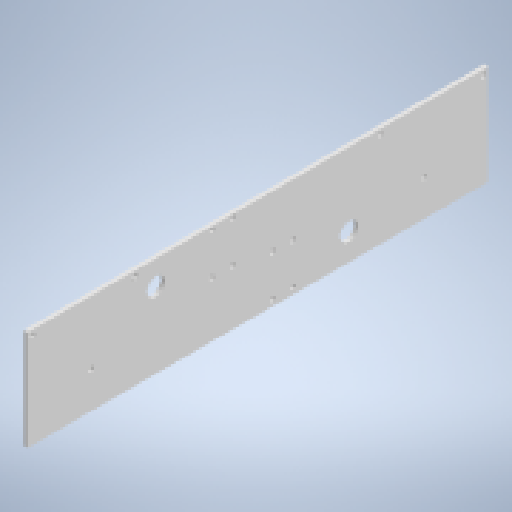
# Autodesk Inventor part: OutsideChassiPlate4.0
Saved by Autodesk Inventor 2023 (Build 270158000, 158)
## iProperties
Created: 2022-09-29
Part Number: OutsideChassiPlate4.0
Material: Generic
Document SubType Name: Modeling
Designer: deli
Density: 1 g/cm^3
Appearance: Default
Author: deli
Autodesk Inventor part; units mm, degrees
ref_plane "YZ Plane" through (0, 0, 0) normal (1, 0, 0) x (0, 1, 0)
ref_plane "XZ Plane" through (0, 0, 0) normal (0, 1, 0) x (-1, 0, 0)
ref_plane "XY Plane" through (0, 0, 0) normal (0, 0, 1) x (1, 0, 0)
sketch "Sketch1" plane through (0, 0, 0) normal (1, 0, 0) x (0, 1, 0)
  line L0 (9.3448, 271.1671) -> (-68.6552, 271.1671)
  line L1 (-68.6552, 271.1671) -> (-68.6552, -93.8329)
  line L2 (-68.6552, -93.8329) -> (9.3448, -93.8329)
  line L3 (9.3448, -93.8329) -> (9.3448, 271.1671)
  circle A0 centre (-40.6552, 221.1671) radius 2
  circle A1 centre (-40.6552, -43.8329) radius 2
  circle A2 centre (-40.6552, 221.1671) radius 48 construction
  circle A3 centre (-40.6552, -43.8329) radius 48 construction
  circle A4 centre (5.3448, 267.1671) radius 2
  circle A5 centre (6.2948, 113.5225) radius 1.9844
  circle A6 centre (6.2948, 97.5225) radius 1.9844
  circle A7 centre (-25.7052, 97.5225) radius 1.9844
  circle A8 centre (-25.7052, 113.5225) radius 1.9844
  line L4 (6.2948, 113.5225) -> (6.2948, 97.5225) construction
  line L5 (6.2948, 97.5225) -> (-25.7052, 97.5225) construction
  line L6 (-25.7052, 97.5225) -> (-25.7052, 113.5225) construction
  line L7 (-25.7052, 113.5225) -> (6.2948, 113.5225) construction
  line L8 (9.3448, 120.2535) -> (-28.7552, 120.2535) construction
  line L9 (-28.7552, 120.2535) -> (-28.7552, 80.5025) construction
  line L10 (-28.7552, 80.5025) -> (9.3448, 80.5025) construction
  line L11 (9.3448, 80.5025) -> (9.3448, 120.2535) construction
  line L12 (7.5668, 120.2535) -> (-26.9772, 120.2535) construction
  line L13 (-26.9772, 120.2535) -> (-26.9772, 129.5255) construction
  line L14 (-26.9772, 129.5255) -> (7.5668, 129.5255) construction
  line L15 (7.5668, 129.5255) -> (7.5668, 120.2535) construction
  line L16 (-4.3712, 129.5255) -> (-15.0392, 129.5255) construction
  line L17 (-15.0392, 129.5255) -> (-15.0392, 137.5255) construction
  line L18 (-15.0392, 137.5255) -> (-4.3712, 137.5255) construction
  line L19 (-4.3712, 137.5255) -> (-4.3712, 129.5255) construction
  line L20 (-5.7052, 137.5255) -> (-13.7052, 137.5255) construction
  line L21 (-13.7052, 137.5255) -> (-13.7052, 140.5255) construction
  line L22 (-13.7052, 140.5255) -> (-5.7052, 140.5255) construction
  line L23 (-5.7052, 140.5255) -> (-5.7052, 137.5255) construction
  line L24 (9.2948, 80.5025) -> (-28.7052, 80.5025) construction
  line L25 (-28.7052, 80.5025) -> (-28.7052, 5.5025) construction
  line L26 (-28.7052, 5.5025) -> (9.2948, 5.5025) construction
  line L27 (9.2948, 5.5025) -> (9.2948, 80.5025) construction
  line L28 (-0.1552, 158.5255) -> (-19.2552, 158.5255) construction
  line L29 (-19.2552, 158.5255) -> (-20.7052, 154.2297) construction
  line L30 (1.2948, 154.2297) -> (-0.1552, 158.5255) construction
  line L31 (1.2948, 140.5255) -> (-20.7052, 140.5255) construction
  line L32 (-20.7052, 140.5255) -> (-20.7052, 154.2297) construction
  line L33 (-20.7052, 154.2297) -> (1.2948, 154.2297) construction
  line L34 (1.2948, 154.2297) -> (1.2948, 140.5255) construction
  line L35 (-20.7052, 154.2297) -> (1.2948, 154.2297) construction
  circle A9 centre (-9.7052, 165.0782) radius 11 construction
  circle A10 centre (-9.7052, 165.0782) radius 7
  circle A11 centre (-9.7052, 165.0782) radius 12.7324 construction
  circle A12 centre (-40.6552, 221.1671) radius 11.9366 construction
  line L36 (-30.2766, 227.0634) -> (1.3653, 171.3676) construction
  line L37 (-20.9286, 159.0658) -> (-51.1772, 215.5304) construction
  circle A13 centre (-65.6052, 63.5958) radius 1.9844
  circle A14 centre (-65.6052, 79.5958) radius 1.9844
  circle A15 centre (-33.6052, 79.5958) radius 1.9844
  circle A16 centre (-33.6052, 63.5958) radius 1.9844
  line L38 (-65.6052, 63.5958) -> (-65.6052, 79.5958) construction
  line L39 (-65.6052, 79.5958) -> (-33.6052, 79.5958) construction
  line L40 (-33.6052, 79.5958) -> (-33.6052, 63.5958) construction
  line L41 (-33.6052, 63.5958) -> (-65.6052, 63.5958) construction
  line L42 (-68.6552, 56.8648) -> (-30.5552, 56.8648) construction
  line L43 (-30.5552, 56.8648) -> (-30.5552, 96.6158) construction
  line L44 (-30.5552, 96.6158) -> (-68.6552, 96.6158) construction
  line L45 (-68.6552, 96.6158) -> (-68.6552, 56.8648) construction
  line L46 (-66.8772, 56.8648) -> (-32.3332, 56.8648) construction
  line L47 (-32.3332, 56.8648) -> (-32.3332, 47.5928) construction
  line L48 (-32.3332, 47.5928) -> (-66.8772, 47.5928) construction
  line L49 (-66.8772, 47.5928) -> (-66.8772, 56.8648) construction
  line L50 (-54.9392, 47.5928) -> (-44.2712, 47.5928) construction
  line L51 (-44.2712, 47.5928) -> (-44.2712, 39.5928) construction
  line L52 (-44.2712, 39.5928) -> (-54.9392, 39.5928) construction
  line L53 (-54.9392, 39.5928) -> (-54.9392, 47.5928) construction
  line L54 (-53.6052, 39.5928) -> (-45.6052, 39.5928) construction
  line L55 (-45.6052, 39.5928) -> (-45.6052, 36.5928) construction
  line L56 (-45.6052, 36.5928) -> (-53.6052, 36.5928) construction
  line L57 (-53.6052, 36.5928) -> (-53.6052, 39.5928) construction
  line L58 (-68.6052, 96.6158) -> (-30.6052, 96.6158) construction
  line L59 (-30.6052, 96.6158) -> (-30.6052, 171.6158) construction
  line L60 (-30.6052, 171.6158) -> (-68.6052, 171.6158) construction
  line L61 (-68.6052, 171.6158) -> (-68.6052, 96.6158) construction
  line L62 (-56.4632, 26.4582) -> (-42.7472, 26.4582) construction
  line L63 (-42.7472, 26.4582) -> (-39.4452, 30.2428) construction
  line L64 (-59.7652, 30.2428) -> (-56.4632, 26.4582) construction
  line L65 (-55.8282, 36.5928) -> (-43.3822, 36.5928) construction
  line L66 (-43.3822, 36.5928) -> (-43.3822, 30.2428) construction
  line L67 (-43.3822, 30.2428) -> (-55.8282, 30.2428) construction
  line L68 (-55.8282, 30.2428) -> (-55.8282, 36.5928) construction
  line L69 (-39.4452, 30.2428) -> (-59.7652, 30.2428) construction
  circle A17 centre (-49.6052, 19.6002) radius 10.16 construction
  circle A18 centre (-49.6052, 19.6002) radius 7
  circle A19 centre (-49.6052, 19.6002) radius 12.7324 construction
  circle A20 centre (-40.6552, -43.8329) radius 11.9366 construction
  line L70 (-36.9766, 21.2223) -> (-28.8159, -42.3122) construction
  line L71 (-52.4532, -45.6473) -> (-62.1897, 17.6649) construction
  circle A21 centre (5.3448, -89.8329) radius 2
  circle A22 centre (5.3448, 187.1671) radius 2
  circle A23 centre (5.3448, -9.8329) radius 2
  point P0 (0, 0)
  point P1 (-50.0041, 6.874)
  point P2 (-48.9722, 32.3168)
  dimension "d0" = 365
  dimension "d1" = 4
  dimension "d2" = 4
  dimension "d3" = 50
  dimension "d4" = 50
  dimension "d5" = 28
  dimension "d6" = 96
  dimension "d7" = 96
  dimension "d8" = 50
  dimension "d9" = 50
  dimension "d10" = 4
  dimension "d11" = 4
  dimension "d12" = 4
  dimension "d13" = 3.9688
  dimension "d14" = 3.9688
  dimension "d15" = 3.9688
  dimension "d16" = 3.9688
  dimension "d17" = 16
  dimension "d18" = 32
  dimension "d19" = 38.1
  dimension "d20" = 3.05
  dimension "d21" = 39.751
  dimension "d22" = 6.731
  dimension "d23" = 34.544
  dimension "d24" = 1.778
  dimension "d25" = 9.272
  dimension "d26" = 10.668
  dimension "d27" = 8
  dimension "d28" = 13.716
  dimension "d29" = 8
  dimension "d30" = 3
  dimension "d32" = 15.05
  dimension "d33" = 38
  dimension "d34" = 0.05
  dimension "d35" = 75
  dimension "d38" = 22
  dimension "d39" = 8.05
  dimension "d42" = 18
  dimension "d45" = 22
  dimension "d46" = 8.05
  dimension "d47" = 19.1
  dimension "d48" = 22
  dimension "d49" = 19.05
  dimension "d50" = 6.5527
  dimension "d51" = 14
  dimension "d52" = 25.4648
  dimension "d53" = 23.8732
  dimension "d54" = 178.576
  dimension "d55" = 178.576
  dimension "d56" = 64.0564
  dimension "d57" = 3.9688
  dimension "d58" = 3.9688
  dimension "d59" = 3.9688
  dimension "d60" = 3.9688
  dimension "d61" = 16
  dimension "d62" = 32
  dimension "d63" = 38.1
  dimension "d64" = 3.05
  dimension "d65" = 39.751
  dimension "d66" = 6.731
  dimension "d67" = 34.544
  dimension "d68" = 1.778
  dimension "d69" = 9.272
  dimension "d70" = 10.668
  constraints: 144 end point, 27 parallel, 24 centre point, 19 perpendicular, 12 point on line, 10 horizontal, 10 point on circle, 8 coincident, 8 tangent, 2 equal length, 2 vertical
  measures "d0" distance of L2.end L0.start
  measures "d1" diameter of A0
  measures "d2" diameter of A1
  measures "d3" distance from line of L3 A0.centre
  measures "d4" distance from line of L3 A1.centre
  measures "d5" distance from line of A0.centre L1
  measures "d6" diameter of A2
  measures "d7" diameter of A3
  measures "d8" distance from line of L0 A2.centre
  measures "d9" distance from line of L2 A1.centre
  measures "d10" diameter of A4
  measures "d11" distance from line of A4.centre L3
  measures "d12" distance from line of L0 A4.centre
  measures "d13" diameter of A5
  measures "d14" diameter of A6
  measures "d15" diameter of A8
  measures "d16" diameter of A7
  measures "d17" distance of L4.start L4.end
  measures "d18" distance of L6.end L4.start
  measures "d19" distance of L10.end L9.end
  measures "d20" distance from line of L4.start L11
  measures "d21" distance of L10.end L8.start
  measures "d22" distance from line of L4.start L8
  measures "d23" distance of L13.end L14.end
  measures "d24" distance between parallel lines of L11 L15
  measures "d25" distance of L14.end L12.start
  measures "d26" distance of L17.end L18.end
  measures "d27" distance of L16.end L17.end
  measures "d28" distance between parallel lines of L11 L19
  measures "d29" distance of L21.end L22.end
  measures "d30" distance of L20.end L21.end
  measures "d32" distance between parallel lines of L11 L23
  measures "d33" distance of L26.end L25.end
  measures "d34" distance between parallel lines of L11 L27
  measures "d35" distance of L26.end L24.start
  measures "d38" distance of L32.end L33.end
  measures "d39" distance between parallel lines of L11 L34
  measures "d42" distance between parallel lines of L31 L28
  measures "d45" distance of L29.end L30.start
  measures "d46" distance from line of L11 L30.start
  measures "d47" distance of L28.start L28.end
  measures "d48" diameter of A9
  measures "d49" distance from line of L11 A9.centre
  measures "d50" distance from line of L28 A9.centre
  measures "d51" diameter of A10
  measures "d52" diameter of A11
  measures "d53" diameter of A12
  measures "d56" distance of L36.start L36.end
  measures "d57" diameter of A13
  measures "d58" diameter of A14
  measures "d59" diameter of A16
  measures "d60" diameter of A15
  measures "d61" distance of L38.start L38.end
  measures "d62" distance of L40.end L38.start
  measures "d63" distance of L44.end L44.start
  measures "d64" distance from line of L38.start L45
  measures "d65" distance of L44.end L42.start
  measures "d66" distance from line of L38.start L42
  measures "d67" distance of L47.end L48.end
  measures "d68" distance between parallel lines of L45 L49
  measures "d69" distance of L48.end L46.start
  measures "d70" distance of L51.end L53.start
extrude "Extrusion1" add sketch "Sketch1" along normal blind 3.175
equation "\"d4\" = d3"
equation "\"d8\" = d3"
equation "\"d9\" = d8"
equation "\"d12\" = d11"
equation "\"d14\" = d13"
equation "\"d15\" = d13"
equation "\"d16\" = d13"
equation "\"d20\" = -0.5 * d18 + 0.5 * d19"
equation "\"d24\" = -0.5 * d23 + 0.5 * d19"
equation "\"d28\" = -0.5 * d26 + 0.5 * d19"
equation "\"d32\" = -0.5 * d29 + 0.5 * d19"
equation "\"d34\" = -0.5 * d33 + 0.5 * d19"
equation "\"d39\" = -0.5 * d38 + 0.5 * d19"
equation "\"d46\" = -0.5 * d45 + 0.5 * d19"
equation "\"d49\" = 0.5 * d19"
body "Solid1"
